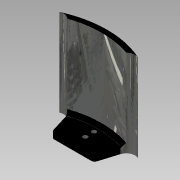
# Autodesk Inventor part: UVTRONwall
Saved by Autodesk Inventor 2015 SP1 (Build 190203100, 203)
## iProperties
Created: 2015-01-28
Part Number: UVTRONwall
Material: Generic
Document SubType Name: Modeling
Designer: Rafi Kurnia Putra
Density: 1 g/cm^3
Appearance: Chrome - Polished
Author: Rafi Kurnia Putra
Autodesk Inventor part; units mm, degrees
ref_plane "YZ Plane" through (0, 0, 0) normal (1, 0, 0) x (0, 1, 0)
ref_plane "XZ Plane" through (0, 0, 0) normal (0, 1, 0) x (-1, 0, 0)
ref_plane "XY Plane" through (0, 0, 0) normal (0, 0, 1) x (1, 0, 0)
sketch "Sketch1" plane through (0, 0, 0) normal (0, 1, 0) x (-1, 0, 0)
  line L0 (12.2682, 17.9043) -> (15.3247, 7.884)
  arc A0 (15.3247, 7.884) -> (22.1712, 4.7888) centre (20.1071, 9.3429) ccw
  arc A1 (-22.1667, 4.7888) -> (-15.3202, 7.884) centre (-20.1027, 9.3429) ccw
  line L1 (-12.2637, 17.9043) -> (-15.3202, 7.884)
  line L2 (10.3552, 19.3208) -> (-10.3507, 19.3208)
  arc A2 (12.2682, 17.9043) -> (10.3552, 19.3208) centre (10.3552, 17.3208) ccw
  arc A3 (-10.3507, 19.3208) -> (-12.2637, 17.9043) centre (-10.3507, 17.3208) ccw
  circle A4 centre (0.0022, 7.3208) radius 1.25
  circle A5 centre (0.0022, 12.3208) radius 1.25
  arc A6 (-22.1667, 4.7888) -> (22.0404, 4.7317) centre (0, 53.698) ccw
  point P0 (0, 0)
  point P1 (28.8757, 53.55)
  point P2 (16.8979, 2.7266)
  point P3 (-28.8757, 53.55)
  point P4 (-16.8934, 2.7266)
  point P5 (-37.9702, 69.5664)
  point P6 (0, 0)
  dimension "d0" = 5
  dimension "d1" = 2
  dimension "d2" = 2.5
  dimension "d3" = 2.5
  dimension "d4" = 34.3772
  dimension "d5" = 1.2868
  dimension "d6" = 1.2911
  dimension "d7" = 5
  dimension "d8" = 7
  dimension "d9" = 20.7059
  dimension "d10" = 10.0203
  dimension "d11" = 10.0203
  dimension "d12" = 13.3613
  dimension "d13" = 14.8201
  dimension "d14" = 53.698
  dimension "d15" = 7.3208
  constraints: 12 point on circle, 7 centre point, 6 end point, 5 tangent, 2 point on line, 1 coincident, 1 equal radius, 1 horizontal
  measures "d0" radius of A0
  measures "d1" radius of A2
  measures "d2" diameter of A4
  measures "d3" diameter of A5
  measures "d4" distance from line of L2 A6.centre
  measures "d5" distance from line of L1 A6.centre
  measures "d6" distance from line of L0 A6.centre
  measures "d7" distance of A4.centre A5.centre
  measures "d8" distance from line of L2 A5.centre
  measures "d9" distance of L2.start L2.end
  measures "d10" vertical distance of L0.start L0.end
  measures "d11" vertical distance of L1.start L1.end
  measures "d12" distance from line of L1 A5.centre
  measures "d13" distance from line of L0 A4.centre
  measures "d14" radius of A6
  measures "d15" distance of A4.centre point (0, 0)
extrude "Extrusion1" add sketch "Sketch1" along normal blind 3
sketch "Sketch2" plane through (0, 3, 0) normal (0, 1, 0) x (1, 0, 0)
  arc A0 (22.1667, -4.7888) -> (16.585, -5.7895) centre (20.1027, -9.3429) ccw
  arc A1 (22.1667, -4.7888) -> (-22.0404, -4.7317) centre (0, -53.698) ccw
  arc A2 (-16.5884, -5.7907) -> (-22.0404, -4.7317) centre (-20.1071, -9.3429) ccw
  line L0 (9.3019, -15.6178) -> (9.24, -15.8208)
  line L1 (-9.2445, -15.8208) -> (-9.3064, -15.6178)
  line L2 (9.24, -15.8208) -> (9.0278, -15.8208)
  line L3 (-9.0323, -15.8208) -> (-9.2445, -15.8208)
  arc A3 (16.585, -5.7895) -> (-16.5884, -5.7907) centre (0, -53.698) ccw
  point P0 (0, 0)
  dimension "d21" = 3
  constraints: 8 end point, 8 point on circle, 7 centre point, 1 other
  measures "d21" radial gap between concentric circles of A1 A3
extrude "Extrusion2" add sketch "Sketch2" along normal blind 46
sketch "Sketch3" plane through (0, 3, 0) normal (0, 1, 0) x (1, 0, 0)
  arc A0 (16.585, -5.7895) -> (-16.5884, -5.7907) centre (0, -53.698) ccw projected
  arc A1 (15.4832, -7.4296) -> (-15.4871, -7.4309) centre (0, -53.698) ccw
  arc A2 (16.585, -5.7895) -> (15.3202, -7.884) centre (20.1027, -9.3429) ccw projected
  arc A3 (-15.3247, -7.884) -> (-16.5884, -5.7907) centre (-20.1071, -9.3429) ccw projected
  point P0 (0, 0)
  dimension "d22" = 1.9077
  constraints: 4 point on circle, 1 centre point
  measures "d22" radial gap between concentric circles of A0 A1
extrude "Extrusion3" add sketch "Sketch3" along normal blind 2
chamfer "Chamfer1" distance 1.9 angle 45 1 edges at (-0.0021, 5, 4.9077)
body "Solid1"
